Autodesk Fusion 360 part; units mm, degrees
(part 3 of 3)
extrude "돌출1''''''''''''" add sketch "스케치3 (8)" along normal blind 82.382 separate body makes body 15 in component "leftPalmRest2"
sketch "스케치1 (12)" plane through (0, 0, -15) normal (0, 0, -1) x (1, 0, 0) in component "leftPalmRest2"
  line L0 (-82.382, 40) -> (-87.382, 40)
  line L1 (-87.382, 40) -> (-87.382, 49)
  line L2 (-85.382, 47) -> (-85.382, 42)
  line L3 (-85.382, 42) -> (-82.382, 42)
  line L4 (-82.382, 47) -> (-85.382, 47)
  line L5 (-87.382, 49) -> (-82.382, 49)
  line L6 (-82.382, 40) -> (-87.382, 40)
  line L7 (-87.382, 49) -> (-87.382, 40)
  line L8 (-87.382, 49) -> (-82.382, 49)
  line L9 (-82.382, 47) -> (-82.382, 49)
  line L10 (-82.382, 47) -> (-85.382, 47)
  line L11 (-85.382, 47) -> (-85.382, 42)
  line L12 (-85.382, 42) -> (-82.382, 42)
  line L13 (-82.382, 42) -> (-82.382, 40)
  constraint coincident L0.start L6.start
  constraint coincident L0.end L1.start
  constraint coincident L1.end L5.start
  constraint coincident L5.end L8.end
  constraint coincident L4.start L9.start
  constraint coincident L2.start L4.end
  constraint coincident L2.end L3.start
  constraint coincident L3.end L12.end
extrude "돌출2'''''''''''" add sketch "스케치2 (10)" against normal blind 3 contours L0 L1 L2 L3 L4 L5 L6 L7 L8 L9 L10 L11 L12 bodies 15 in component "leftPalmRest2"
draft "기울기1'" angle -10 neutral plane through (-82.382, -10, -15) pull (0, 0.99999, 0.004531) 1 faces at (0, -51.9908, -9) on bodies 15 in component "leftPalmRest2"
fillet "모깎기1''''''''" radius 5 5 edges at (-161.1171, -33.0269, 3) (-119.7266, -55.9723, 3) (-154.0689, -72.9862, 0) (-151.0618, -90, -9) (-116.7243, -90, -3) on bodies 14 in component "leftPalmRest"
fillet "모깎기1'''''''''" radius 5 5 edges at (-4.0458, -33.0269, 3) (-45.2368, -55.9723, 3) (-11.0941, -72.9862, 0) (-48.2392, -90, -3) (-14.1012, -90, -9) on bodies 15 in component "leftPalmRest2"
component "leftKey1" placed x (1, 0, 0) y (0, 1, 0) z (0, 0, 1) at (0, 0, 0)
component "leftKey2" placed x (1, 0, 0) y (0, 1, 0) z (0, 0, 1) at (0, 0, 0)
component "leftBody1" placed x (1, 0, 0) y (0, 1, 0) z (0, 0, 1) at (0, 0, 0)
component "leftBody2" placed x (1, 0, 0) y (0, 1, 0) z (0, 0, 1) at (0, 0, 0)
component "rightKey1" placed x (1, 0, 0) y (0, 1, 0) z (0, 0, 1) at (0, 0, 0)
component "rightKey2" placed x (1, 0, 0) y (0, 1, 0) z (0, 0, 1) at (0, 0, 0)
component "rightBody1" placed x (1, 0, 0) y (0, 1, 0) z (0, 0, 1) at (0, 0, 0)
component "rightBody2" placed x (1, 0, 0) y (0, 1, 0) z (0, 0, 1) at (0, 0, 0)
component "tempJoin" placed x (1, 0, 0) y (0, 1, 0) z (0, 0, 1) at (13.5824, 154.2275, -3.4182)
component "rightPalmRest1" placed x (1, 0, 0) y (0, 1, 0) z (0, 0, 1) at (0, 0, 0)
component "rightPalmRest2" placed x (1, 0, 0) y (0, 1, 0) z (0, 0, 1) at (0, 0, 0)
component "leftPalmRest" placed x (1, 0, 0) y (0, 1, 0) z (0, 0, 1) at (0, 0, 0)
component "leftPalmRest2" placed x (1, 0, 0) y (0, 1, 0) z (0, 0, 1) at (0, 0, 0)
equation "keyHoleWidth = 14 mm"
equation "keyWidth = 19.05 mm"
equation "bodyMargin = 4 mm"
equation "boltKeyHole = 3.2 mm"
equation "boltBodyHole = 3 mm"
equation "d6 = boltKeyHole"
equation "bodyBoltCenterMargin = 3.1 mm"
equation "d8 = bodyBoltCenterMargin"
equation "d9 = bodyBoltCenterMargin"
equation "boltHead = 6 mm"
equation "d12 = boltKeyHole"
equation "d14 = bodyBoltCenterMargin"
equation "d15 = bodyBoltCenterMargin"
equation "d16 = ( 1.25 * 4 * keyWidth ) + ( 2.25 * keyWidth ) + bodyMargin"
equation "d17 = ( 5 * keyWidth ) + bodyMargin * 2"
equation "d18 = keyHoleWidth"
equation "d19 = keyHoleWidth"
equation "keyMargin = ( keyWidth - keyHoleWidth ) / 2"
equation "d21 = ( keyWidth * 1.25 - keyHoleWidth ) / 2"
equation "d22 = bodyMargin + keyMargin"
equation "d25 = keyWidth * 1.25"
equation "d32 = keyHoleWidth"
equation "d33 = keyHoleWidth"
equation "d37 = keyWidth"
equation "d39 = keyHoleWidth"
equation "d40 = keyHoleWidth"
equation "d41 = ( keyWidth * 1.75 - keyHoleWidth ) / 2"
equation "d43 = keyHoleWidth"
equation "d44 = keyHoleWidth"
equation "d45 = ( keyWidth * 1.75 - keyHoleWidth ) / 2 + keyMargin"
equation "d48 = keyWidth"
equation "d50 = keyHoleWidth"
equation "d51 = keyHoleWidth"
equation "d52 = ( keyWidth * 1.5 - keyHoleWidth ) / 2"
equation "d53 = keyWidth"
equation "d54 = keyHoleWidth"
equation "d55 = keyHoleWidth"
equation "d56 = ( keyWidth * 1.5 - keyHoleWidth ) / 2 + keyMargin"
equation "d59 = keyWidth"
equation "d61 = keyHoleWidth"
equation "d62 = keyHoleWidth"
equation "d64 = keyMargin"
equation "d68 = keyWidth"
equation "d70 = keyWidth"
equation "d71 = boltKeyHole"
equation "d73 = bodyBoltCenterMargin"
equation "d74 = boltKeyHole"
equation "d82 = width"
equation "d83 = width"
equation "d85 = stabilHeight"
equation "d87 = ( stabilHeight - 2.2 mm ) / 2"
equation "d88 = ( keyHoleWidth - 2.2 mm ) / 2"
equation "d89 = ( keyWidth * 1.25 - keyHoleWidth ) / 2 + ( keyWidth * 2.25 - keyHoleWidth ) / 2"
equation "d90 = width"
equation "d91 = width"
equation "d93 = stabilHeight"
equation "d95 = ( stabilHeight - 2.2 mm ) / 2"
equation "d96 = ( keyHoleWidth - 2.2 mm ) / 2"
equation "d97 = keyWidth"
equation "d98 = ( keyWidth * 2.25 - keyHoleWidth ) / 2"
equation "d99 = keyWidth"
equation "d100 = ( keyWidth * 2.25 - keyHoleWidth ) / 2 + keyMargin"
equation "d101 = keyPlateHeight"
equation "d103 = boltHead"
equation "d104 = boltHead"
equation "d105 = boltHead"
equation "d106 = boltHead"
equation "d107 = -boltHeadDepth"
equation "d109 = keyWidth + bodyMargin"
equation "d110 = keyWidth * 5 + bodyMargin * 2"
equation "d111 = keyHoleWidth"
equation "d112 = keyHoleWidth"
equation "d113 = bodyMargin + keyMargin"
equation "d114 = keyMargin"
equation "d118 = keyWidth"
equation "d119 = bodyBoltCenterMargin"
equation "d120 = bodyBoltCenterMargin"
equation "d121 = bodyBoltCenterMargin"
equation "d122 = boltKeyHole"
equation "d123 = bodyBoltCenterMargin"
equation "d124 = boltKeyHole"
equation "d125 = bodyBoltCenterMargin"
equation "d126 = boltKeyHole"
equation "d127 = keyPlateHeight"
equation "d129 = boltHead"
equation "d130 = boltHead"
equation "d131 = boltHead"
equation "d132 = boltHead"
equation "boltHeadDepth = 1.75 mm"
equation "d134 = -boltHeadDepth"
equation "d136 = ( keyWidth + ( 1.25 * 4 * keyWidth ) + ( 2.25 * keyWidth ) + bodyMargin * 2 ) / 2"
equation "d137 = boltBodyHole"
equation "d138 = boltBodyHole"
equation "d139 = boltBodyHole"
equation "d140 = boltBodyHole"
equation "d141 = boltBodyHole"
equation "d142 = bodyBoltMargin"
equation "bodyBoltMargin = 4.75 mm"
equation "bodyWallDepth = 2.5 mm"
equation "d145 = bodyBoltMargin"
equation "d146 = bodyBoltMargin"
equation "d147 = bodyBoltMargin"
equation "d149 = bodyWallDepth"
equation "d151 = bodyWallDepth"
equation "d152 = bodyWallDepth"
equation "d153 = bodyWallDepth"
equation "bodyHeight = 15 mm"
equation "bodyDepth = bodyHeight - 2 mm"
equation "d156 = -bodyHeight"
equation "d158 = -bodyDepth"
equation "bodyBoltHoleDepth = bodyDepth - 3 mm"
equation "d161 = -bodyBoltHoleDepth"
equation "d163 = ( keyWidth + ( 1.25 * 4 * keyWidth ) + ( 2.25 * keyWidth ) + bodyMargin * 2 ) / 2"
equation "d164 = keyWidth * 5 + bodyMargin * 2"
equation "d165 = boltBodyHole"
equation "d166 = boltBodyHole"
equation "d167 = boltBodyHole"
equation "d168 = boltBodyHole"
equation "d169 = boltBodyHole"
equation "d170 = boltBodyHole"
equation "d171 = boltBodyHole"
equation "d172 = bodyBoltCenterMargin"
equation "d173 = boltBodyHole"
equation "d174 = bodyBoltCenterMargin"
equation "d175 = bodyBoltMargin"
equation "d176 = bodyBoltMargin"
equation "d177 = bodyBoltMargin"
equation "d178 = bodyBoltMargin"
equation "d179 = bodyBoltMargin"
equation "d180 = bodyBoltMargin"
equation "d181 = bodyBoltMargin"
equation "d182 = bodyBoltMargin"
equation "d183 = bodyWallDepth"
equation "d185 = bodyWallDepth"
equation "d186 = bodyWallDepth"
equation "d187 = bodyWallDepth"
equation "d189 = bodyWallDepth"
equation "d190 = -bodyHeight"
equation "d192 = -bodyDepth"
equation "d194 = -bodyBoltHoleDepth"
equation "d196 = ( keyWidth + ( 1.25 * 4 * keyWidth ) + ( 2.25 * keyWidth ) + bodyMargin * 2 ) / 2"
equation "d197 = boltKeyHole"
equation "d198 = bodyBoltCenterMargin"
equation "d199 = boltKeyHole"
equation "d200 = bodyBoltCenterMargin"
equation "d201 = boltKeyHole"
equation "d202 = boltKeyHole"
equation "d203 = bodyBoltCenterMargin"
equation "d204 = bodyBoltCenterMargin"
equation "d205 = boltHead"
equation "d206 = boltHead"
equation "d207 = boltHead"
equation "d208 = boltHead"
equation "d210 = roundRadios"
equation "roundRadios = 3.1 mm"
equation "d217 = roundRadios"
equation "keyPlateHeight = 3 mm"
equation "d222 = roundRadios"
equation "d242 = ( ( 18 - ( 5.8 ) ) / 2 ) * 1 mm"
equation "d245 = -bodyWallDepth"
equation "d247 = -bodyWallDepth + 1 mm"
equation "d386 = keyWidth * 5 + bodyMargin * 2"
equation "d392 = width"
equation "d393 = width"
equation "d395 = stabilHeight"
equation "d397 = ( stabilHeight - 2.2 mm ) / 2"
equation "d398 = ( keyHoleWidth - 2.2 mm ) / 2"
equation "d400 = keyHoleWidth"
equation "d401 = keyHoleWidth"
equation "d402 = ( keyWidth * 2.75 - keyHoleWidth ) / 2 + keyMargin"
equation "d443 = boltKeyHole"
equation "d448 = boltKeyHole"
equation "d449 = bodyBoltCenterMargin"
equation "d450 = boltKeyHole"
equation "d451 = bodyBoltCenterMargin"
equation "d491 = keyHoleWidth"
equation "d492 = keyHoleWidth"
equation "d493 = keyMargin + keyWidth + bodyMargin"
equation "d494 = keyMargin + bodyMargin"
equation "d506 = keyHoleWidth"
equation "d507 = keyHoleWidth"
equation "d508 = keyWidth"
equation "d509 = keyHoleWidth"
equation "d510 = keyHoleWidth"
equation "d511 = ( keyWidth * 1.75 - keyHoleWidth ) / 2 + keyMargin"
equation "d512 = keyHoleWidth"
equation "d513 = keyHoleWidth"
equation "d514 = ( keyWidth * 1.75 - keyHoleWidth ) / 2 + keyMargin"
equation "d515 = width"
equation "d516 = width"
equation "d518 = stabilHeight"
equation "d520 = ( stabilHeight - 2.2 mm ) / 2"
equation "d521 = ( keyHoleWidth - 2.2 mm ) / 2"
equation "d522 = keyWidth"
equation "d523 = ( keyWidth * 2.25 - keyHoleWidth ) / 2 + keyWidth + bodyMargin"
equation "d524 = keyHoleWidth"
equation "d525 = keyHoleWidth"
equation "d526 = ( keyWidth * 2.25 - keyHoleWidth ) / 2 + keyMargin"
equation "d527 = keyHoleWidth"
equation "d528 = keyHoleWidth"
equation "d529 = keyWidth"
equation "d530 = ( keyWidth * 1.5 - keyHoleWidth ) / 2 + keyWidth + bodyMargin"
equation "d531 = keyHoleWidth"
equation "d532 = keyHoleWidth"
equation "d533 = ( keyWidth * 1.5 - keyHoleWidth ) / 2 + keyMargin"
equation "d534 = width"
equation "d535 = width"
equation "d537 = stabilHeight"
equation "d539 = ( stabilHeight - 2.2 mm ) / 2"
equation "d540 = ( keyHoleWidth - 2.2 mm ) / 2"
equation "d541 = keyWidth"
equation "d542 = ( keyWidth * 2 - keyHoleWidth ) / 2 + keyWidth + bodyMargin"
equation "d543 = keyHoleWidth"
equation "d544 = keyHoleWidth"
equation "d545 = ( keyWidth * 2 - keyHoleWidth ) / 2 + keyMargin"
equation "d546 = boltKeyHole"
equation "d547 = bodyBoltCenterMargin"
equation "d548 = bodyBoltCenterMargin"
equation "d549 = boltKeyHole"
equation "d550 = bodyBoltCenterMargin"
equation "d555 = keyHoleWidth"
equation "d556 = keyHoleWidth"
equation "d557 = keyMargin + bodyMargin"
equation "d570 = keyHoleWidth"
equation "d571 = keyHoleWidth"
equation "d573 = keyWidth"
equation "d574 = keyWidth"
equation "d575 = keyWidth"
equation "d579 = keyHoleWidth"
equation "d580 = keyHoleWidth"
equation "d581 = keyHoleWidth"
equation "d582 = keyHoleWidth"
equation "d583 = keyHoleWidth"
equation "d584 = keyHoleWidth"
equation "d587 = keyWidth"
equation "d591 = keyWidth"
equation "d595 = keyWidth"
equation "d599 = keyWidth"
equation "d604 = bodyBoltCenterMargin"
equation "d605 = boltKeyHole"
equation "d606 = bodyBoltCenterMargin"
equation "d607 = bodyBoltCenterMargin"
equation "d608 = boltKeyHole"
equation "d609 = bodyBoltCenterMargin"
equation "d610 = bodyBoltCenterMargin"
equation "d614 = boltHead"
equation "d615 = boltHead"
equation "d616 = boltHead"
equation "d617 = boltHead"
equation "d618 = -boltHeadDepth"
equation "d621 = roundRadios"
equation "d622 = bodyMargin * 2 + ( keyWidth * 8 ) + keyWidth * 2 + 30 mm"
equation "d625 = boltKeyHole"
equation "d626 = bodyBoltCenterMargin"
equation "d627 = boltKeyHole"
equation "d628 = boltKeyHole"
equation "d629 = bodyBoltCenterMargin"
equation "d630 = bodyBoltCenterMargin"
equation "d631 = boltKeyHole"
equation "d632 = boltKeyHole"
equation "d633 = boltKeyHole"
equation "d634 = bodyBoltCenterMargin"
equation "d637 = bodyBoltCenterMargin"
equation "d639 = keyPlateHeight"
equation "d641 = boltHead"
equation "d642 = boltHead"
equation "d643 = boltHead"
equation "d644 = boltHead"
equation "d645 = boltHead"
equation "d646 = boltHead"
equation "d647 = boltHead"
equation "d649 = boltHead"
equation "d650 = -boltHeadDepth"
equation "d653 = roundRadios"
equation "d654 = keyPlateHeight"
equation "d656 = boltHead"
equation "d657 = boltHead"
equation "d658 = boltHead"
equation "d659 = boltHead"
equation "d660 = -boltHeadDepth"
equation "d663 = roundRadios"
equation "d664 = boltBodyHole"
equation "d665 = boltBodyHole"
equation "d666 = boltBodyHole"
equation "d667 = boltBodyHole"
equation "d668 = boltBodyHole"
equation "d669 = boltBodyHole"
equation "d670 = boltBodyHole"
equation "d671 = boltBodyHole"
equation "d672 = bodyBoltMargin"
equation "d674 = bodyBoltMargin"
equation "d675 = bodyBoltMargin"
equation "d676 = bodyBoltMargin"
equation "d677 = bodyBoltMargin"
equation "d678 = bodyBoltMargin"
equation "d679 = bodyBoltMargin"
equation "d680 = bodyWallDepth"
equation "d682 = bodyWallDepth"
equation "d683 = bodyWallDepth"
equation "d686 = bodyBoltMargin"
equation "d687 = bodyWallDepth"
equation "d688 = bodyWallDepth"
equation "d689 = bodyWallDepth"
equation "d690 = bodyWallDepth"
equation "d691 = -bodyHeight"
equation "d693 = -bodyDepth"
equation "d695 = -bodyBoltHoleDepth"
equation "d699 = boltBodyHole"
equation "d700 = boltBodyHole"
equation "d701 = boltBodyHole"
equation "d702 = boltBodyHole"
equation "d703 = bodyBoltMargin"
equation "d704 = bodyBoltMargin"
equation "d705 = bodyBoltMargin"
equation "d706 = bodyBoltMargin"
equation "d707 = bodyWallDepth"
equation "d708 = bodyWallDepth"
equation "d710 = bodyWallDepth"
equation "d711 = bodyWallDepth"
equation "d712 = -bodyHeight"
equation "d714 = -bodyDepth"
equation "d716 = -bodyBoltHoleDepth"
equation "d735 = ( 3.6 / 2 ) * 1 mm"
equation "d739 = -bodyWallDepth"
equation "d741 = -bodyWallDepth + 1 mm"
equation "d743 = bodyBoltMargin"
equation "d744 = boltBodyHole"
equation "d745 = boltBodyHole"
equation "d749 = roundRadios"
equation "d751 = roundRadios"
equation "d753 = bodyDepth"
equation "d756 = bodyDepth"
equation "d759 = roundRadios"
equation "stabilHeight = 11.2 mm"
equation "d767 = bodyDepth"
equation "d773 = bodyDepth"
equation "d777 = bodyHeight + keyPlateHeight"
